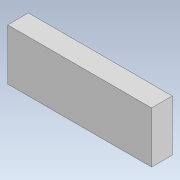
# Autodesk Inventor part: Блок питания MA-60-12_12V
Saved by Autodesk Inventor 2021.2 (Build 252289000, 289)
## iProperties
Created: 2022-11-29
Part Number: Блок питания MA-60-12_12V
Material: Типовые
Document SubType Name: Modeling
Designer: Voodoo
Mass: 159.432 g
Surface Area: 235 cm^2
Volume: 159.432 cm^3
Density: 1 g/cm^3
Appearance: По умолчанию
Author: Voodoo
Autodesk Inventor part; units mm, degrees
ref_plane "YZ Plane" through (0, 0, 0) normal (1, 0, 0) x (0, 1, 0)
ref_plane "XZ Plane" through (0, 0, 0) normal (0, 1, 0) x (-1, 0, 0)
ref_plane "XY Plane" through (0, 0, 0) normal (0, 0, 1) x (1, 0, 0)
sketch "Эскиз1" plane through (0, 0, 0) normal (0, 0, 1) x (1, 0, 0)
  line L0 (-73, -26) -> (73, -26)
  line L1 (73, -26) -> (73, 26)
  line L2 (73, 26) -> (-73, 26)
  line L3 (-73, 26) -> (-73, -26)
  line L4 (-73, -26) -> (73, 26) construction
  line L5 (73, -26) -> (-73, 26) construction
  point P0 (0, 0)
  dimension "d0" = 146
  dimension "d1" = 52
  constraints: 12 end point, 2 midpoint, 2 parallel, 1 horizontal, 1 perpendicular
  measures "d0" distance of L1.end L2.end
  measures "d1" distance of L2.end L0.start
extrude "Выдавливание1" add sketch "Эскиз1" along normal blind 21
